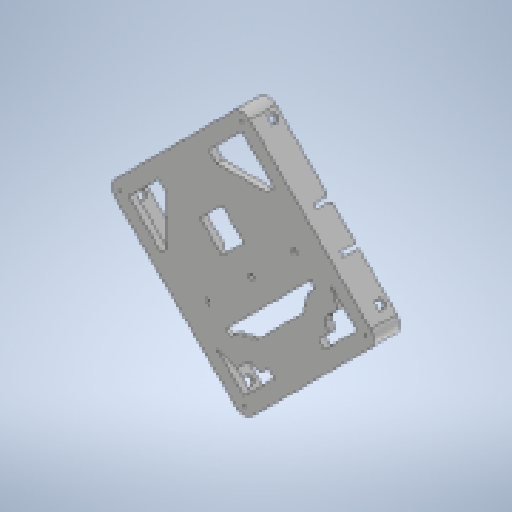
# Autodesk Inventor part: RobotStandBase
Saved by Autodesk Inventor 2025.1 (Build 291241000, 241)
## iProperties
Created: 2026-05-10
Part Number: RobotStandBase
Material: Generic
Document SubType Name: Modeling
Designer: User
Density: 1 g/cm^3
Appearance: Default
Author: User
## iProperties of the stored document RobotStandBase_3DPrint.ipt
Created: 2026-05-10
Part Number: RobotStandBase_3DPrint
Material: Generic
Document SubType Name: Modeling
Designer: User
Density: 1 g/cm^3
Appearance: Default
Author: User
Autodesk Inventor part; units mm, degrees
(part 1 of 2)
ref_plane "YZ Plane" through (0, 0, 0) normal (1, 0, 0) x (0, 1, 0)
ref_plane "XZ Plane" through (0, 0, 0) normal (0, 1, 0) x (-1, 0, 0)
ref_plane "XY Plane" through (0, 0, 0) normal (0, 0, 1) x (1, 0, 0)
sketch "Sketch1" plane through (0, 0, 0) normal (0, 0, 1) x (1, 0, 0)
  line L0 (-56.2755, 56.2755) -> (-1.1212, 1.1212) projected
  line L1 (-1.1163, -113.435) -> (-56.398, -168.7168) projected
  line L2 (-167.8767, -165.6343) -> (-223.031, -110.4799) projected
  line L3 (-226.1086, 0.9938) -> (-170.8268, 56.2755) projected
  line L4 (-280.3067, -53.2043) -> (-226.1086, 0.9938)
  line L5 (-280.3067, -53.2043) -> (-223.031, -110.4799)
  line L6 (-170.8268, 56.2755) -> (-113.5512, 113.5512)
  line L7 (-113.5512, 113.5512) -> (-56.2755, 56.2755)
  line L8 (-1.1212, 1.1212) -> (56.1594, -56.1594)
  line L9 (56.1594, -56.1594) -> (-1.1163, -113.435)
  line L10 (-167.8767, -165.6343) -> (-110.5961, -222.9149)
  line L11 (-56.398, -168.7168) -> (-110.5961, -222.9149)
  point P0 (0, 0)
  constraints: 16 end point, 4 point on line, 2 perpendicular, 1 collinear
extrude "Extrusion1" add sketch "Sketch1" along normal blind 5
sketch "Sketch2" plane through (0, 0, 0) normal (0, 0, -1) x (-1, 0, 0)
  line L0 (-56.1594, -56.1594) -> (113.5512, 113.5512) projected
  line L1 (-52.6239, -59.6949) -> (117.0867, 110.0157)
  line L2 (113.5512, 113.5512) -> (280.3067, -53.2043) projected
  line L3 (110.5961, -222.9149) -> (-56.1594, -56.1594) projected
  point P0 (0, 0)
  dimension "d2" = 5
  constraints: 2 end point, 1 parallel
  measures "d2" distance between parallel lines of L0 L1
ref_plane "Work Plane1" through (-173.6553, -9.9637, -27.5) normal (0, 0, 1) x (1, 0, 0)
extrude "Extrusion2" add sketch "Sketch2" along normal up to surface (27.5 mm away)
sketch "Sketch3" plane through (-113.5512, 113.5512, -27.5) normal (0.7071068, 0.7071068, 0) x (-0.7071068, 0.7071068, 0)
  line L0 (-106.0221, 0) -> (-106.0221, 18.3301) projected
  line L1 (-111.0221, 18.3301) -> (-111.0221, 0) projected
  line L2 (-106.0221, 18.3301) -> (-111.0221, 18.3301) projected
  line L3 (-154, 0) -> (-154, 18.3301) projected
  line L4 (-159, 18.3301) -> (-159, -12) projected
  line L5 (-154, 18.3301) -> (-159, 18.3301) projected
  line L6 (-111.2221, 0) -> (-111.2221, 18.5301)
  line L7 (-111.2221, 18.5301) -> (-105.8221, 18.5301)
  line L8 (-105.8221, 18.5301) -> (-105.8221, 0)
  line L9 (-153.8, 0) -> (-153.8, 18.5301)
  line L10 (-153.8, 18.5301) -> (-159.2, 18.5301)
  line L11 (-159.2, 18.5301) -> (-159.2, -12)
  line L12 (0, 0) -> (-240.007, 0) projected
  point P0 (-160.5856, 27.5)
  point P1 (-159.2, 0)
  dimension "d5" = 0.2
  dimension "d6" = 0.2
  constraints: 12 end point, 4 other
  measures "d5" distance between parallel lines of L1 L6
  measures "d6" distance between parallel lines of L3 L9
extrude "Extrusion3" cut sketch "Sketch3" against normal blind 10
sketch "Sketch4" plane through (0, 0, 0) normal (0, 0, -1) x (-1, 0, 0)
  line L0 (280.3067, -53.2043) -> (110.5961, -222.9149) projected
  line L1 (276.7711, -49.6687) -> (107.0605, -219.3793)
  line L2 (107.0605, -219.3793) -> (110.5961, -222.9149)
  line L3 (117.0867, 110.0157) -> (280.3067, -53.2043) projected
  line L4 (276.7711, -49.6687) -> (280.3067, -53.2043)
  line L5 (110.5961, -222.9149) -> (-52.6239, -59.6949) projected
  point P0 (0, 0)
  dimension "d9" = 5
  constraints: 6 end point, 1 collinear, 1 parallel
  measures "d9" distance between parallel lines of L0 L1
ref_plane "Work Plane2" through (-226.1086, -128.1732, -27.5) normal (0, 0, 1) x (1, 0, 0)
extrude "Extrusion4" add sketch "Sketch4" along normal up to surface (27.5 mm away)
sketch "Sketch5" plane through (-110.5961, -222.9149, 5) normal (-0.7071068, -0.7071068, 0) x (-0.7071068, 0.7071068, 0)
  line L0 (81.007, 14.1699) -> (81.007, 44.5) projected
  line L1 (86.007, 14.1699) -> (86.007, 32.5) projected
  line L2 (81.007, 14.1699) -> (86.007, 14.1699) projected
  line L3 (128.9849, 32.5) -> (128.9849, 14.1699) projected
  line L4 (128.9849, 14.1699) -> (133.9849, 14.1699) projected
  line L5 (133.9849, 14.1699) -> (133.9849, 32.5) projected
  line L6 (86.207, 32.5) -> (86.207, 13.9699)
  line L7 (86.207, 13.9699) -> (80.807, 13.9699)
  line L8 (80.807, 13.9699) -> (80.807, 44.5)
  line L9 (128.7849, 32.5) -> (128.7849, 13.9699)
  line L10 (128.7849, 13.9699) -> (134.1849, 13.9699)
  line L11 (134.1849, 13.9699) -> (134.1849, 32.5)
  line L12 (0, 32.5) -> (240.007, 32.5) projected
  point P0 (79.4214, 5)
  point P1 (80.807, 32.5)
  dimension "d12" = 0.2
  dimension "d13" = 0.2
  constraints: 12 end point, 4 other
  measures "d12" distance between parallel lines of L1 L6
  measures "d13" distance between parallel lines of L3 L9
extrude "Extrusion5" cut sketch "Sketch5" against normal blind 10
sketch "Sketch6" plane through (0, 0, 0) normal (0, 0, -1) x (-1, 0, 0)
  line L0 (107.0605, -219.3793) -> (-52.6239, -59.6949) projected
  line L1 (110.5961, -215.8438) -> (-49.0883, -56.1594)
  line L2 (117.0867, 110.0157) -> (-52.6239, -59.6949) projected
  line L3 (107.0605, -219.3793) -> (276.7711, -49.6687) projected
  point P0 (0, 0)
  dimension "d16" = 5
  constraints: 2 end point, 1 parallel
  measures "d16" distance between parallel lines of L0 L1
extrude "Extrusion6" add sketch "Sketch6" along normal up to surface (27.5 mm away)
sketch "Sketch7" plane through (56.1594, -56.1594, 5) normal (0.7071068, -0.7071068, 0) x (-0.7071068, -0.7071068, 0)
  line L0 (91, 32.5) -> (91, 14.1699) projected
  line L1 (96, 14.1699) -> (96, 32.5) projected
  line L2 (91, 14.1699) -> (96, 14.1699) projected
  line L3 (144.1802, 32.5) -> (144.1802, 14.1699) projected
  line L4 (144.1802, 14.1699) -> (149.1802, 14.1699) projected
  line L5 (149.1802, 14.1699) -> (149.1802, 32.5) projected
  line L6 (90.8, 32.5) -> (90.8, 13.9699)
  line L7 (90.8, 13.9699) -> (96.2, 13.9699)
  line L8 (96.2, 13.9699) -> (96.2, 32.5)
  line L9 (143.9802, 32.5) -> (143.9802, 13.9699)
  line L10 (143.9802, 13.9699) -> (149.3802, 13.9699)
  line L11 (149.3802, 13.9699) -> (149.3802, 32.5)
  line L12 (0, 32.5) -> (235.8278, 32.5) projected
  point P0 (0, 5)
  dimension "d19" = 0.2
  dimension "d20" = 0.2
  constraints: 12 end point, 5 other
  measures "d19" distance between parallel lines of L0 L6
  measures "d20" distance between parallel lines of L3 L9
extrude "Extrusion7" cut sketch "Sketch7" against normal blind 10
sketch "Sketch8" plane through (0, 0, 0) normal (0, 0, -1) x (-1, 0, 0)
  line L0 (117.0867, 110.0157) -> (276.7711, -49.6687) projected
  line L1 (113.5512, 106.4801) -> (273.2356, -53.2043)
  line L2 (117.0867, 110.0157) -> (-49.0883, -56.1594) projected
  line L3 (110.5961, -215.8438) -> (276.7711, -49.6687) projected
  point P0 (0, 0)
  dimension "d23" = 5
  constraints: 2 end point, 1 parallel
  measures "d23" distance between parallel lines of L0 L1
extrude "Extrusion8" add sketch "Sketch8" along normal up to surface (27.5 mm away)
sketch "Sketch9" plane through (-280.3067, -53.2043, -27.5) normal (-0.7071068, 0.7071068, 0) x (-0.7071068, -0.7071068, 0)
  line L0 (-139.8278, 0) -> (-139.8278, 18.3301) projected
  line L1 (-150.8278, 0) -> (-144.8278, 6) projected
  line L2 (-144.8278, 18.3301) -> (-144.8278, 6) projected
  line L3 (-139.8278, 18.3301) -> (-144.8278, 18.3301) projected
  line L4 (-91.6476, 18.3301) -> (-91.6476, 0) projected
  line L5 (-86.6476, 6) -> (-80.6476, 0) projected
  line L6 (-86.6476, 6) -> (-86.6476, 18.3301) projected
  line L7 (-86.6476, 18.3301) -> (-91.6476, 18.3301) projected
  line L8 (-91.8476, 0) -> (-91.8476, 18.5301)
  line L9 (-91.8476, 18.5301) -> (-86.4476, 18.5301)
  line L10 (-86.4476, 18.5301) -> (-86.4476, 6.0828)
  line L11 (-86.4476, 6.0828) -> (-80.5062, 0.1414)
  line L12 (-139.6278, 0) -> (-139.6278, 18.5301)
  line L13 (-139.6278, 18.5301) -> (-145.0278, 18.5301)
  line L14 (-145.0278, 18.5301) -> (-145.0278, 6.0828)
  line L15 (-145.0278, 6.0828) -> (-150.9693, 0.1414)
  line L16 (-230.8278, 0) -> (-5, 0) projected
  line L17 (-145.0278, 6.0828) -> (-151.1107, 0)
  line L18 (-86.4476, 6.0828) -> (-80.3648, 0)
  point P0 (-235.8278, 27.5)
  point P1 (-150.9693, 0.1414)
  point P2 (-80.5062, 0.1414)
  dimension "d26" = 0.2
  dimension "d27" = 0.2
  constraints: 20 end point, 2 point on line, 9 other
  measures "d26" distance between parallel lines of L4 L8
  measures "d27" distance between parallel lines of L0 L12
extrude "Extrusion9" cut sketch "Sketch9" against normal blind 10
chamfer "Chamfer1" distance 2 angle 45 16 edges at (-221.7124, 1.8544, -27.5) (-213.5928, 9.974, -27.5) (-179.8071, 43.7597, -27.5) (-171.6875, 51.8793, -27.5) (-36.673, 33.1375, -27.5) (-40.4914, 36.9559, -27.5) (-6.5659, 3.0304, -27.5) (-2.7476, -0.788, -27.5) (-13.632, -122.4153, -27.5) (-9.8137, -118.5969, -27.5) (-47.4178, -156.201, -27.5) (-51.2361, -160.0194, -27.5) (-165.9675, -164.0079, -27.5) (-169.7859, -160.1895, -27.5) (-199.893, -130.0824, -27.5) (-203.7113, -126.2641, -27.5)
fillet "Fillet1" radius 9 4 edges at (49.0883, -56.1594, -13.75) (-273.2356, -53.2043, -13.75) (-113.5512, 106.4801, -13.75) (-110.5961, -215.8438, -13.75)
fillet "Fillet2" radius 14 4 edges at (-110.5961, -222.9149, -11.25) (-280.3067, -53.2043, -11.25) (56.1594, -56.1594, -11.25) (-113.5512, 113.5512, -11.25)
chamfer "Chamfer2" distance 9 angle 45 8 edges at (-32.2314, 25.1604, 0) (45.3604, -56.1594, 0) (-30.7539, -136.0016, 0) (-110.5961, -212.1159, 0) (-191.9158, -134.524, 0) (-269.5077, -53.2043, 0) (-193.3934, 26.6379, 0) (-113.5512, 102.7522, 0)
sketch "Sketch10" plane through (-38.4408, 31.3697, -9) normal (-0.7071068, -0.7071068, 0) x (-0.7071068, 0.7071068, 0)
  line L0 (-42.5779, 16.5) -> (-42.5779, 0) projected
  line L1 (-47.9779, 0) -> (-47.9779, 16.5) projected
  line L2 (-49.9779, 18.5) -> (-47.9779, 16.5) projected
  line L3 (-42.5779, 16.5) -> (-40.5779, 18.5) projected
  line L4 (-40.5779, 18.5) -> (-2, 18.5) projected
  line L5 (-114.7849, 18.5) -> (-49.9779, 18.5) projected
  line L6 (-42.5779, -0.0301) -> (-47.9779, -0.0301) projected
  line L7 (-2, 18.5) -> (0, 16.5) projected
  line L8 (5.4, 16.5) -> (7.4, 18.5) projected
  line L9 (7.4, 18.5) -> (97.2221, 18.5) projected
  line L10 (5.4, 16.5) -> (5.4, 0) projected
  line L11 (5.4, -0.0301) -> (0, -0.0301) projected
  line L12 (0, 0) -> (0, 16.5) projected
  line L13 (-3, 0) -> (-3, 15.2574)
  line L14 (-3, 15.2574) -> (-3.2426, 15.5)
  line L15 (-3.2426, 15.5) -> (-39.3352, 15.5)
  line L16 (-39.3352, 15.5) -> (-39.5779, 15.2574)
  line L17 (-39.5779, 15.2574) -> (-39.5779, 0)
  line L18 (-50.9779, 0) -> (-50.9779, 15.2574)
  line L19 (-50.9779, 15.2574) -> (-51.2205, 15.5)
  line L20 (-51.2205, 15.5) -> (-114.7849, 15.5)
  line L21 (8.4, 0) -> (8.4, 15.2574)
  line L22 (8.4, 15.2574) -> (8.6426, 15.5)
  line L23 (8.6426, 15.5) -> (97.2221, 15.5)
  line L24 (-39.5779, 18.5) -> (-39.5779, 0)
  line L25 (0, 0) -> (-42.5779, 0) projected
  line L26 (-39.5779, 0) -> (-39.5779, -3)
  line L27 (-39.5779, -3) -> (-50.9779, -3)
  line L28 (-50.9779, -3) -> (-50.9779, 18.5)
  line L29 (-3, 18.5) -> (-3, 0)
  line L30 (-3, 0) -> (-3, -3)
  line L31 (-3, 0) -> (0, 0) construction
  line L32 (-3, -3) -> (8.4, -3)
  line L33 (8.4, -3) -> (8.4, 18.5)
  line L34 (5.4, -0.0301) -> (5.4, 0) projected
  line L35 (0, 0) -> (0, -0.0301) projected
  line L36 (-47.9779, 0) -> (-47.9779, -0.0301) projected
  line L37 (-42.5779, -0.0301) -> (-42.5779, 0) projected
  point P0 (-49.3635, -9)
  point P1 (-3, 15.2574)
  point P2 (8.4, 0)
  point P3 (8.4, 15.2574)
  point P4 (-50.9779, 15.2574)
  point P5 (-50.9779, 0)
  point P6 (-39.5779, 15.2574)
  dimension "d174" = 1
  dimension "d38" = 3
  dimension "d39" = 3
  dimension "d40" = 3
  dimension "d41" = 3
  dimension "d42" = 90
  dimension "d43" = 3
  dimension "d44" = 90
  dimension "d45" = 90
  constraints: 40 end point, 7 point on line, 2 perpendicular, 1 collinear, 1 horizontal, 1 vertical, 8 other
  measures "d38" distance between parallel lines of L12 L13
  measures "d39" distance between parallel lines of L1 L18
  measures "d40" distance between parallel lines of L10 L21
  measures "d41" distance of L17.end L26.end
  measures "d42" angle of L26 L27
  measures "d43" distance of L13.start L30.end
  measures "d44" angle of L30 L31
  measures "d45" angle of L32 L30
extrude "Extrusion10" add sketch "Sketch10" along normal blind 3 contours L3 L4 L24 L17 L25 L0 | L25 L26 L27 L28 L18 L5 L2 L1 L36 L6 L37 | L13 L29 L4 L7 L12 L25 | L25 L35 L11 L34 L10 L8 L9 L33 L21 L32 L30
sketch "Sketch11" plane through (-49.4684, -161.7872, -8.9699) normal (0.7071068, -0.7071068, 0) x (-0.7071068, -0.7071068, 0)
  line L0 (-135.3802, -13.9699) -> (-135.3802, 18.5301) projected
  line L1 (72.4476, -13.9699) -> (-135.3802, -13.9699) projected
  line L2 (72.4476, 18.5301) -> (72.4476, -13.9699) projected
  line L3 (2, 18.5301) -> (72.4476, 18.5301) projected
  line L4 (0, 16.5301) -> (2, 18.5301) projected
  line L5 (0, 16.5301) -> (0, 0) projected
  line L6 (0, 0) -> (-5.4, 0) projected
  line L7 (-5.4, 0) -> (-5.4, 16.5301) projected
  line L8 (-7.4, 18.5301) -> (-5.4, 16.5301) projected
  line L9 (-51.1802, 18.5301) -> (-7.4, 18.5301) projected
  line L10 (-53.1802, 16.5301) -> (-51.1802, 18.5301) projected
  line L11 (-53.1802, 16.5301) -> (-53.1802, 0) projected
  line L12 (-53.1802, 0) -> (-58.5802, 0) projected
  line L13 (-58.5802, 0) -> (-58.5802, 16.5301) projected
  line L14 (-60.5802, 18.5301) -> (-58.5802, 16.5301) projected
  line L15 (-135.3802, 18.5301) -> (-60.5802, 18.5301) projected
  line L16 (-61.8229, 15.5301) -> (-61.5802, 15.2875)
  line L17 (-61.5802, 15.2875) -> (-61.5802, -3)
  line L18 (-61.5802, -3) -> (-50.1802, -3)
  line L19 (-50.1802, -3) -> (-50.1802, 15.2875)
  line L20 (-50.1802, 15.2875) -> (-49.9376, 15.5301)
  line L21 (-49.9376, 15.5301) -> (-8.6426, 15.5301)
  line L22 (-8.6426, 15.5301) -> (-8.4, 15.2875)
  line L23 (-8.4, 15.2875) -> (-8.4, -3)
  line L24 (-8.4, -3) -> (3, -3)
  line L25 (3, -3) -> (3, 15.2875)
  line L26 (3, 15.2875) -> (3.2426, 15.5301)
  line L27 (3.2426, 15.5301) -> (69.4476, 15.5301)
  line L28 (69.4476, 15.5301) -> (69.4476, -10.9699)
  line L29 (69.4476, -10.9699) -> (-132.3802, -10.9699)
  line L30 (-132.3802, -10.9699) -> (-132.3802, 15.5301)
  line L31 (-132.3802, 15.5301) -> (-61.8229, 15.5301)
  line L32 (-61.5802, -3) -> (-61.5802, 18.5301)
  line L33 (-50.1802, -3) -> (-50.1802, 18.5301)
  line L34 (-51.1802, 18.5301) -> (-7.4, 18.5301) projected
  line L35 (-8.4, -3) -> (-8.4, 18.5301)
  line L36 (3, -3) -> (3, 18.5301)
  point P0 (-149.3802, -8.9699)
  point P1 (-8.4, 15.2875)
  point P2 (3, 15.2875)
  point P3 (-61.5802, 15.2875)
  point P4 (-50.1802, 15.2875)
  point P5 (-50.1802, 18.5301)
  dimension "d48" = 3
  constraints: 40 end point, 4 point on line, 2 parallel, 1 perpendicular, 1 vertical, 15 other
  measures "d48" distance between parallel lines of L15 L31
extrude "Extrusion11" add sketch "Sketch11" against normal blind 8 contours L15 L14 L13 L12 L11 L10 L9 L33 L19 L18 L17 L32 | L36 L25 L24 L23 L35 L9 L8 L7 L6 L5 L4 L3
sketch "Sketch12" plane through (-205.4791, -128.0318, -8.9699) normal (-0.7071068, -0.7071068, 0) x (-0.7071068, 0.7071068, 0)
  line L0 (91.8221, 18.5301) -> (91.8221, -13.9699) projected
  line L1 (2, 18.5301) -> (91.8221, 18.5301) projected
  line L2 (0, 16.5301) -> (2, 18.5301) projected
  line L3 (0, 16.5301) -> (0, 0) projected
  line L4 (0, 0) -> (-5.4, 0) projected
  line L5 (-5.4, 0) -> (-5.4, 16.5301) projected
  line L6 (-7.4, 18.5301) -> (-5.4, 16.5301) projected
  line L7 (-45.9779, 18.5301) -> (-7.4, 18.5301) projected
  line L8 (-47.9779, 16.5301) -> (-45.9779, 18.5301) projected
  line L9 (-47.9779, 16.5301) -> (-47.9779, 0) projected
  line L10 (-47.9779, 0) -> (-53.3779, 0) projected
  line L11 (-53.3779, 0) -> (-53.3779, 16.5301) projected
  line L12 (-55.3779, 18.5301) -> (-53.3779, 16.5301) projected
  line L13 (-120.1849, 18.5301) -> (-55.3779, 18.5301) projected
  line L14 (-120.1849, -13.9699) -> (-120.1849, 18.5301) projected
  line L15 (91.8221, -13.9699) -> (-120.1849, -13.9699) projected
  line L16 (-8.4, 15.2875) -> (-8.4, -3)
  line L17 (-8.4, -3) -> (3, -3)
  line L18 (3, -3) -> (3, 15.2875)
  line L19 (3, 15.2875) -> (3.2426, 15.5301)
  line L20 (3.2426, 15.5301) -> (88.8221, 15.5301)
  line L21 (88.8221, 15.5301) -> (88.8221, -10.9699)
  line L22 (88.8221, -10.9699) -> (-117.1849, -10.9699)
  line L23 (-117.1849, -10.9699) -> (-117.1849, 15.5301)
  line L24 (-117.1849, 15.5301) -> (-56.6205, 15.5301)
  line L25 (-56.6205, 15.5301) -> (-56.3779, 15.2875)
  line L26 (-56.3779, 15.2875) -> (-56.3779, -3)
  line L27 (-56.3779, -3) -> (-44.9779, -3)
  line L28 (-44.9779, -3) -> (-44.9779, 15.2875)
  line L29 (-44.9779, 15.2875) -> (-44.7352, 15.5301)
  line L30 (-44.7352, 15.5301) -> (-8.6426, 15.5301)
  line L31 (-8.6426, 15.5301) -> (-8.4, 15.2875)
  line L32 (3, 18.5301) -> (3, 0.0301) projected
  line L33 (3, -3) -> (3, 18.5301)
  line L34 (-8.4, -3) -> (-8.4, 18.5301)
  line L35 (-44.9779, 0.0301) -> (-44.9779, -2.9699) projected
  line L36 (-44.9779, 18.5301) -> (-44.9779, 0.0301) projected
  line L37 (-44.9779, -2.9699) -> (-44.9779, 18.5301)
  line L38 (-56.3779, -3) -> (-56.3779, 18.5301)
  point P0 (-54.7635, -8.9699)
  point P1 (-56.3779, 15.2875)
  point P2 (-8.4, 15.2875)
  dimension "d51" = 3
  constraints: 40 end point, 3 point on line, 1 collinear, 1 perpendicular, 15 other
  measures "d51" distance between parallel lines of L5 L16
extrude "Extrusion12" add sketch "Sketch12" against normal blind 8 contours L32 L18 L17 L16 L34 L7 L6 L5 L4 L3 L2 L1 | L13 L12 L11 L10 L9 L8 L7 L36 L28 L27 L26 L38
sketch "Sketch13" plane through (-177.7565, 49.3459, -21.4172) normal (-0.7071068, 0.7071068, 0) x (-0.7071068, -0.7071068, 0)
  line L0 (-76.8, -6.0828) -> (-76.8, 26.4172) projected
  line L1 (-8.0828, -6.0828) -> (-76.8, -6.0828) projected
  line L2 (-4.6686, -4.6686) -> (-8.0828, -6.0828) projected
  line L3 (-4.6686, -4.6686) -> (0, 0) projected
  line L4 (0, 0) -> (0, 12.4473) projected
  line L5 (0, 12.4473) -> (5.4, 12.4473) projected
  line L6 (5.4, 12.4473) -> (5.4, -4.0828) projected
  line L7 (7.4, -6.0828) -> (5.4, -4.0828) projected
  line L8 (51.1802, -6.0828) -> (7.4, -6.0828) projected
  line L9 (53.1802, -4.0828) -> (51.1802, -6.0828) projected
  line L10 (53.1802, -4.0828) -> (53.1802, 12.4473) projected
  line L11 (53.1802, 12.4473) -> (58.5802, 12.4473) projected
  line L12 (58.5802, 12.4473) -> (58.5802, 0) projected
  line L13 (58.5802, 0) -> (63.2489, -4.6686) projected
  line L14 (66.6631, -6.0828) -> (63.2489, -4.6686) projected
  line L15 (131.0278, -6.0828) -> (66.6631, -6.0828) projected
  line L16 (131.0278, 26.4172) -> (131.0278, -6.0828) projected
  line L17 (-76.8, 26.4172) -> (131.0278, 26.4172) projected
  line L18 (8.6426, -3.0828) -> (8.4, -2.8402)
  line L19 (8.4, -2.8402) -> (8.4, 15.4473)
  line L20 (8.4, 15.4473) -> (-3, 15.4473)
  line L21 (-3, 15.4473) -> (-3, 1.2426)
  line L22 (-3, 1.2426) -> (-6.368, -2.1254)
  line L23 (-6.368, -2.1254) -> (-8.6796, -3.0828)
  line L24 (-8.6796, -3.0828) -> (-73.8, -3.0828)
  line L25 (-73.8, -3.0828) -> (-73.8, 23.4172)
  line L26 (-73.8, 23.4172) -> (128.0278, 23.4172)
  line L27 (128.0278, 23.4172) -> (128.0278, -3.0828)
  line L28 (128.0278, -3.0828) -> (67.2598, -3.0828)
  line L29 (67.2598, -3.0828) -> (64.9482, -2.1254)
  line L30 (64.9482, -2.1254) -> (61.5802, 1.2426)
  line L31 (61.5802, 1.2426) -> (61.5802, 15.4473)
  line L32 (61.5802, 15.4473) -> (50.1802, 15.4473)
  line L33 (50.1802, 15.4473) -> (50.1802, -2.8402)
  line L34 (50.1802, -2.8402) -> (49.9376, -3.0828)
  line L35 (49.9376, -3.0828) -> (8.6426, -3.0828)
  line L36 (50.1802, 15.4172) -> (50.1802, -6.0828) projected
  line L37 (50.1802, 15.4473) -> (50.1802, -6.0828)
  line L38 (8.4, -6.0828) -> (8.4, 15.4172) projected
  line L39 (8.4, 15.4473) -> (8.4, -6.0828)
  line L40 (-8.6796, -3.0828) -> (-8.6796, -6.0828)
  line L41 (67.2598, -3.0828) -> (67.2598, -6.0828)
  point P0 (-90.8, 21.4172)
  dimension "d54" = 3
  constraints: 44 end point, 2 point on line, 1 parallel, 1 perpendicular, 17 other
  measures "d54" distance between parallel lines of L8 L35
extrude "Extrusion13" add sketch "Sketch13" against normal blind 8 contours L40 L23 L22 L21 L20 L19 L38 L8 L7 L6 L5 L4 L3 L2 L1 | L15 L14 L13 L12 L11 L10 L9 L8 L36 L33 L32 L31 L30 L29 L41
sketch "Sketch14" plane through (0, 0, 0) normal (0, 0, -1) x (-1, 0, 0)
  line L0 (168.0234, -127.9604) -> (169.6482, -127.3987) projected
  line L1 (169.6482, -127.3987) -> (173.5542, -123.4928) projected
  line L2 (173.5542, -123.4928) -> (171.3554, -97.3754) projected
  line L3 (171.3554, -97.3754) -> (171.5721, -97.1586) projected
  line L4 (69.9473, 4.4661) -> (171.5721, -97.1586) projected
  line L5 (69.9473, 4.4661) -> (40.9763, 6.9046) projected
  line L6 (40.9763, 6.9046) -> (37.0674, 2.9956) projected
  line L7 (37.0674, 2.9956) -> (27.3005, -25.3557) projected
  line L8 (27.3005, -25.3557) -> (27.2484, -25.4078) projected
  line L9 (27.2484, -25.4078) -> (139.62, -137.7795) projected
  line L10 (139.62, -137.7795) -> (139.6721, -137.7273) projected
  line L11 (139.6721, -137.7273) -> (168.0234, -127.9604) projected
  line L12 (139.6721, -137.7273) -> (171.5721, -97.1586)
  line L13 (27.2484, -25.4078) -> (69.9473, 4.4661)
  line L14 (83.4342, -81.5936) -> (119.7206, -45.3072)
  circle A0 centre (155.6221, -117.443) radius 1.5
  circle A1 centre (101.5774, -63.4504) radius 1.5
  circle A2 centre (48.5978, -10.4708) radius 1.5
  circle A3 centre (48.5978, -10.4708) radius 1.5 projected
  circle A4 centre (101.5774, -63.4504) radius 1.5 projected
  circle A5 centre (155.6221, -117.443) radius 1.5 projected
  point P0 (0, 0)
  dimension "d57" = 3
  dimension "d58" = 3
  dimension "d59" = 3
  constraints: 6 end point, 4 midpoint, 3 centre point, 1 perpendicular, 1 point on line
  measures "d57" diameter of A0
  measures "d58" diameter of A1
  measures "d59" diameter of A2
extrude "Extrusion14" cut sketch "Sketch14" against normal blind 8 contours A0 L12 | L12 A0 | A1 L14 | L14 A1 | A2 L13 | L13 A2
sketch "Sketch15" plane through (0, 0, 5) normal (0, 0, 1) x (1, 0, 0)
  circle A0 centre (-48.5978, -10.4708) radius 1.5 projected
  circle A1 centre (-101.5774, -63.4504) radius 1.5 projected
  circle A2 centre (-155.6221, -117.443) radius 1.5 projected
  circle A3 centre (-155.6221, -117.443) radius 3.25
  circle A4 centre (-101.5774, -63.4504) radius 3.25
  circle A5 centre (-48.5978, -10.4708) radius 1.5 projected
  circle A6 centre (-48.5978, -10.4708) radius 3.25
  point P0 (0, 0)
  dimension "d62" = 6.5
  dimension "d63" = 6.5
  dimension "d64" = 6.5
  constraints: 3 centre point, 3 coincident
  measures "d62" diameter of A3
  measures "d63" diameter of A4
  measures "d64" diameter of A6
extrude "Extrusion15" cut sketch "Sketch15" against normal blind 3
sketch "Sketch16" plane through (-110.5961, -203.1159, -27.5) normal (0, 0, -1) x (-1, 0, 0)
  line L0 (51.4823, 38.7544) -> (6.364, -6.364) projected
  arc A0 (-6.364, -6.364) -> (6.364, -6.364) centre (0, 0) ccw projected
  line L1 (-6.364, -6.364) -> (-55.4708, 42.7429) projected
  line L2 (-55.4708, 42.7429) -> (-53.3495, 44.8642) projected
  line L3 (-54.0566, 45.5713) -> (-53.3495, 44.8642) projected
  line L4 (-59.7135, 39.9145) -> (-54.0566, 45.5713) projected
  line L5 (-59.7135, 39.9145) -> (-9.8995, -9.8995) projected
  arc A1 (-9.8995, -9.8995) -> (9.8995, -9.8995) centre (0, 0) ccw projected
  line L6 (9.8995, -9.8995) -> (55.725, 35.926) projected
  line L7 (55.725, 35.926) -> (50.0681, 41.5828) projected
  line L8 (49.361, 40.8757) -> (50.0681, 41.5828) projected
  line L9 (51.4823, 38.7544) -> (49.361, 40.8757) projected
  line L10 (-29.8223, 58.7748) -> (-54.198, 34.3991) projected
  line L11 (-45.5575, 38.7969) -> (-51.3488, 33.0057) projected
  line L12 (-44.8504, 38.0898) -> (-50.6417, 32.2986)
  line L13 (-50.6625, 37.9346) -> (-47.8341, 35.1062)
  line L14 (-47.8341, 35.1062) -> (-51.3696, 31.5706)
  line L15 (-51.3696, 31.5706) -> (-54.198, 34.3991)
  line L16 (-54.198, 34.3991) -> (-50.6625, 37.9346)
  line L17 (-85.1041, 114.0566) -> (-109.4798, 89.6808) projected
  line L18 (-95.7821, 107.6212) -> (-107.3585, 96.0448) projected
  line L19 (-101.136, 88.408) -> (-153.3204, 140.5925) projected
  line L20 (-156.856, 137.057) -> (-103.9644, 84.1654) projected
  line L21 (-107.3585, 96.0448) -> (-111.6011, 91.8021) projected
  line L22 (-112.3082, 92.5093) -> (-108.0656, 96.7519)
  line L23 (-108.0656, 96.7519) -> (-96.4892, 108.3283)
  line L24 (-108.7727, 96.0448) -> (-105.9443, 93.2164)
  line L25 (-105.9443, 93.2164) -> (-109.4798, 89.6808)
  line L26 (-109.4798, 89.6808) -> (-112.3082, 92.5093)
  line L27 (-112.3082, 92.5093) -> (-108.7727, 96.0448)
  point P0 (-110.5961, 203.1159)
  point P1 (-50.6417, 32.2986)
  point P2 (-112.3082, 92.5093)
  dimension "d67" = 1
  dimension "d68" = 1
  constraints: 22 end point, 8 point on line, 5 parallel, 2 perpendicular, 1 other
  measures "d67" distance between parallel lines of L11 L12
  measures "d68" distance between parallel lines of L21 L22
extrude "Extrusion16" cut sketch "Sketch16" against normal blind 2 contours L12 L14 L5 L10 L1 | L17 L20 L21 L19 | L21 L20 L22 L19
sketch "Sketch17" plane through (-205.4791, -128.0318, -8.9699) normal (-0.7071068, -0.7071068, 0) x (-0.7071068, 0.7071068, 0)
  arc A0 (78.6963, 12.5301) -> (86.9479, 12.5301) centre (82.8221, 9.3651) ccw projected
  circle A1 centre (82.8221, 9.3651) radius 5.2
  arc A2 (-100.0531, 9.3651) -> (-110.4531, 9.3651) centre (-105.2531, 9.3651) ccw projected
  point P0 (-54.7635, -8.9699)
  point P1 (86.9479, 12.5301)
  point P2 (78.6963, 12.5301)
  constraints: 1 centre point, 1 coincident, 1 concentric
extrude "Extrusion17" cut sketch "Sketch17" against normal through all
sketch "Sketch18" plane through (-205.4791, -128.0318, -8.9699) normal (-0.7071068, -0.7071068, 0) x (-0.7071068, 0.7071068, 0)
  circle A0 centre (-105.2531, 9.3651) radius 5.2 projected
  circle A1 centre (82.8221, 9.3651) radius 5.2 projected
  line L0 (77.6221, 4.1651) -> (88.0221, 4.1651)
  line L1 (88.0221, 4.1651) -> (88.0221, 9.3651)
  line L2 (77.6221, 4.1651) -> (77.6221, 9.3651)
  line L3 (-110.4531, 4.1651) -> (-100.0531, 4.1651)
  line L4 (-100.0531, 4.1651) -> (-100.0531, 9.3651)
  line L5 (-110.4531, 4.1651) -> (-110.4531, 9.3651)
  point P0 (-54.7635, -8.9699)
  point P1 (82.8221, 4.1651)
  point P2 (-105.2531, 4.1651)
  constraints: 12 end point, 4 point on circle, 3 tangent, 2 horizontal, 1 parallel
extrude "Extrusion18" cut sketch "Sketch18" against normal through all contours A0 | L4 L3 A0 | A0 L3 L5 | L1 L0 A1 | A1 L0 L2
sketch "Sketch19" plane through (0, 0, 0) normal (0, 0, -1) x (-1, 0, 0)
  line L0 (80.6463, 31.9048) -> (146.4561, 31.9048)
  line L1 (146.4561, 31.9048) -> (165.8771, 51.3258)
  line L2 (80.6463, 31.9048) -> (61.2253, 51.3258)
  line L3 (-36.3604, -56.1594) -> (113.5512, 93.7522) projected
  line L4 (113.5512, 93.7522) -> (260.5077, -53.2043) projected
  line L5 (201.6104, -23.5044) -> (221.1589, -3.956)
  line L6 (201.6104, -23.5044) -> (201.6104, -89.0593)
  line L7 (201.6104, -89.0593) -> (218.0813, -105.5302)
  line L8 (260.5077, -53.2043) -> (110.5961, -203.1159) projected
  line L9 (80.7737, -144.3411) -> (61.3478, -163.7671)
  line L10 (87.6903, -151.2576) -> (80.7737, -144.3411)
  line L11 (87.6903, -151.2576) -> (91.6237, -155.191)
  line L12 (91.6237, -155.191) -> (101.5016, -151.7881)
  line L13 (101.5016, -151.7881) -> (107.3644, -153.2088)
  line L14 (107.3644, -153.2088) -> (108.0393, -153.3992)
  ellipse E0 centre (95.5108, -186.7522) end of major axis (150.7623, -199.5036) minor radius 35.4384 (110.2496, -154.0628) -> (108.0393, -153.3992) ccw
  line L15 (121.0834, -164.8966) -> (110.2496, -154.0628)
  line L16 (143.4515, -157.164) -> (121.0834, -164.8966)
  line L17 (143.4515, -157.164) -> (155.3769, -161.0788)
  line L18 (143.4515, -157.164) -> (155.3769, -161.0788)
  line L19 (143.4515, -157.164) -> (155.3769, -161.0788)
  line L20 (110.5961, -203.1159) -> (-36.3604, -56.1594) projected
  line L21 (25.492, -89.0593) -> (6.066, -108.4853)
  line L22 (25.492, -89.0593) -> (15.5994, -79.1667)
  line L23 (11.6681, -75.2354) -> (15.5994, -79.1667)
  line L24 (15.0798, -65.3663) -> (11.6681, -75.2354)
  line L25 (13.6634, -59.5078) -> (15.0798, -65.3663)
  ellipse E1 centre (-19.8987, -71.3426) end of major axis (-32.6095, -16.1319) minor radius 35.4503 (13.4734, -58.8334) -> (12.8115, -56.6247) ccw
  line L26 (12.8115, -56.6247) -> (0.6153, -44.4285)
  line L27 (13.4734, -58.8334) -> (13.6634, -59.5078)
  line L28 (0.6153, -44.4285) -> (8.1231, -22.711)
  line L29 (4.4924, -10.8835) -> (8.1231, -22.711)
  line L30 (221.6168, -101.9946) -> (206.6104, -86.9882)
  line L31 (206.6104, -86.9882) -> (206.6104, -25.5755)
  line L32 (206.6104, -25.5755) -> (224.6944, -7.4915)
  line L33 (162.3416, 54.8613) -> (144.385, 36.9048)
  line L34 (144.385, 36.9048) -> (82.7174, 36.9048)
  line L35 (82.7174, 36.9048) -> (64.7608, 54.8613)
  line L36 (2.5305, -104.9498) -> (18.4209, -89.0593)
  line L37 (18.4209, -89.0593) -> (5.9203, -76.5587)
  line L38 (5.9203, -76.5587) -> (9.8756, -65.1173)
  line L39 (9.8756, -65.1173) -> (8.8254, -60.7736)
  line L40 (8.8254, -60.7736) -> (8.6633, -60.1983)
  line L41 (8.395, -59.2793) -> (-5.1325, -45.7518)
  line L42 (-5.1325, -45.7518) -> (2.8645, -22.6189)
  line L43 (2.8645, -22.6189) -> (-0.2875, -12.3507)
  line L44 (64.8833, -167.3026) -> (80.7737, -151.4122)
  line L45 (80.7737, -151.4122) -> (90.2977, -160.9361)
  line L46 (90.2977, -160.9361) -> (101.7465, -156.9921)
  line L47 (101.7465, -156.9921) -> (106.0961, -158.0462)
  line L48 (106.0961, -158.0462) -> (106.6721, -158.2087)
  line L49 (107.5941, -158.4784) -> (119.7601, -170.6444)
  line L50 (119.7601, -170.6444) -> (145.0852, -161.8896)
  line L51 (141.8921, -161.9145) -> (153.8174, -165.8294)
  line L52 (-29.2893, -56.1594) -> (113.5512, 86.6811)
  line L53 (113.5512, 86.6811) -> (253.4366, -53.2043)
  line L54 (253.4366, -53.2043) -> (110.5961, -196.0448)
  line L55 (110.5961, -196.0448) -> (-29.2893, -56.1594)
  spline S0 degree 3 poles (8.6633, -60.1983) (8.5756, -59.8914) (8.4862, -59.5851) (8.395, -59.2793) knots 0 0 0 0 1 1 1 1
  spline S1 degree 3 poles (106.6721, -158.2087) (106.98, -158.2969) (107.2873, -158.3868) (107.5941, -158.4784) knots 0 0 0 0 1 1 1 1
  point P0 (0, 0)
  point P1 (153.8563, 46.376)
  point P2 (73.2461, 46.376)
  point P3 (213.1315, -93.5094)
  point P4 (216.2091, -15.9768)
  point P5 (73.3686, -158.8173)
  point P6 (144.0258, -162.615)
  point P7 (143.4928, -162.44)
  point P8 (2.1319, -24.7381)
  point P9 (11.0157, -96.4645)
  dimension "d202" = 3
  dimension "d75" = 5
  dimension "d76" = 5
  dimension "d77" = 5
  dimension "d78" = 5
  dimension "d79" = 5
  dimension "d80" = 5
  constraints: 104 end point, 5 parallel, 1 horizontal, 1 vertical, 88 other
  measures "d75" distance between parallel lines of L6 L31
  measures "d76" distance between parallel lines of L0 L34
  measures "d77" distance between parallel lines of L24 L38
  measures "d78" distance between parallel lines of L15 L49
  measures "d79" distance between parallel lines of L17 L51
  measures "d80" distance between parallel lines of L20 L55
extrude "Extrusion19" cut sketch "Sketch19" against normal blind 10 contours L52 L53 L33 L34 L35 | L42 L41 S0 L40 L39 L38 L37 L36 L55 L52 | L53 L54 L30 L31 L32 | L44 L45 L46 L47 L48 S1 L49 L50 L51 L54 L55
sketch "Sketch20" plane through (0, 0, 0) normal (0, 0, -1) x (-1, 0, 0)
  line L0 (215.502, 11.6004) -> (144.8535, -59.0481)
  line L1 (177.8979, 49.2045) -> (107.2494, -21.4441)
  line L2 (181.4334, 45.6689) -> (110.7849, -24.9796)
  line L3 (219.0375, 8.0648) -> (148.389, -62.5837)
  line L4 (107.2494, -21.4441) -> (110.7849, -24.9796)
  line L5 (144.8535, -59.0481) -> (148.389, -62.5837)
  line L6 (174.3624, 52.74) -> (100.1783, -21.4441)
  line L7 (100.1783, -21.4441) -> (110.7849, -32.0507)
  line L8 (110.7849, -32.0507) -> (184.969, 42.1334)
  line L9 (211.9665, 15.1359) -> (137.7824, -59.0481)
  line L10 (137.7824, -59.0481) -> (148.389, -69.6548)
  line L11 (148.389, -69.6548) -> (222.5731, 4.5293)
  line L12 (137.7824, -59.0481) -> (110.7849, -32.0507)
  line L13 (110.7849, -32.0507) -> (137.7824, -5.0532)
  line L14 (137.7824, -5.0532) -> (164.7799, -32.0507)
  line L15 (164.7799, -32.0507) -> (137.7824, -59.0481)
  point P0 (0, 0)
  dimension "d202" = 3
  dimension "d83" = 5
  dimension "d84" = 5
  constraints: 32 end point, 3 equal length, 1 perpendicular, 16 other
  measures "d83" distance between parallel lines of L1 L6
  measures "d84" distance between parallel lines of L0 L9
extrude "Extrusion20" cut sketch "Sketch20" against normal blind 10
sketch "Sketch21" plane through (0, 0, 5) normal (0, 0, 1) x (1, 0, 0)
  arc A0 (-270.4072, -43.3048) -> (-270.4072, -63.1038) centre (-260.5077, -53.2043) ccw projected
  line L0 (-213.1315, -93.5094) -> (-253.4366, -53.2043) projected
  line L1 (-253.4366, -53.2043) -> (-216.2091, -15.9768) projected
  line L2 (-253.4366, -53.2043) -> (-274.5077, -53.2043)
  circle A1 centre (-263.9721, -53.2043) radius 1.5
  line L3 (-153.8563, 46.376) -> (-113.5512, 86.6811) projected
  line L4 (-113.5512, 86.6811) -> (-113.5512, 107.7522)
  arc A2 (-103.6517, 103.6517) -> (-123.4507, 103.6517) centre (-113.5512, 93.7522) ccw projected
  line L5 (-113.5512, 86.6811) -> (-92.4801, 86.6811) construction
  circle A3 centre (-113.5512, 97.2167) radius 1.5
  line L6 (29.2893, -56.1594) -> (-11.0157, -96.4645) projected
  line L7 (-2.1319, -24.7381) -> (29.2893, -56.1594) projected
  arc A4 (46.2599, -66.0589) -> (46.2599, -46.2599) centre (36.3604, -56.1594) ccw projected
  line L8 (29.2893, -56.1594) -> (50.3604, -56.1594)
  circle A5 centre (39.8249, -56.1594) radius 1.5
  line L9 (-110.5961, -196.0448) -> (-144.0258, -162.615) projected
  line L10 (-73.3686, -158.8173) -> (-110.5961, -196.0448) projected
  arc A6 (-120.4956, -213.0154) -> (-100.6966, -213.0154) centre (-110.5961, -203.1159) ccw projected
  line L11 (-110.5961, -196.0448) -> (-110.5961, -217.1159)
  circle A7 centre (-110.5961, -206.5803) radius 1.5
  point P0 (0, 0)
  dimension "d87" = 3
  dimension "d88" = 90
  dimension "d89" = 3
  dimension "d90" = 3
  dimension "d91" = 3
  constraints: 10 end point, 4 centre point, 4 midpoint, 4 point on circle, 1 horizontal, 1 perpendicular
  measures "d87" diameter of A1
  measures "d88" angle of L5 L4
  measures "d89" diameter of A3
  measures "d90" diameter of A5
  measures "d91" diameter of A7
extrude "Extrusion21" cut sketch "Sketch21" against normal through all
sketch "Sketch22" plane through (0, 0, 0) normal (0, 0, -1) x (-1, 0, 0)
  line L0 (2.1319, -24.7381) -> (-5.1325, -45.7518) projected
  line L1 (-5.1325, -45.7518) -> (8.395, -59.2793) projected
  line L2 (8.8254, -60.7736) -> (9.8756, -65.1173) projected
  circle A0 centre (-39.8249, -56.1594) radius 1.5 projected
  circle A1 centre (113.5512, 97.2167) radius 1.5 projected
  circle A2 centre (110.5961, -206.5803) radius 1.5 projected
  circle A3 centre (263.9721, -53.2043) radius 1.5 projected
  line L3 (164.7799, -32.0507) -> (137.7824, -5.0532) projected
  line L4 (137.7824, -5.0532) -> (110.7849, -32.0507) projected
  line L5 (110.7849, -32.0507) -> (137.7824, -59.0481) projected
  line L6 (137.7824, -59.0481) -> (164.7799, -32.0507) projected
  line L7 (213.1315, -93.5094) -> (253.4366, -53.2043) projected
  line L8 (253.4366, -53.2043) -> (216.2091, -15.9768) projected
  line L9 (216.2091, -15.9768) -> (206.6104, -25.5755) projected
  line L10 (206.6104, -25.5755) -> (206.6104, -86.9882) projected
  line L11 (206.6104, -86.9882) -> (213.1315, -93.5094) projected
  line L12 (106.6721, -158.2087) -> (106.0961, -158.0462) projected
  line L13 (106.0961, -158.0462) -> (101.7465, -156.9921) projected
  line L14 (101.7465, -156.9921) -> (90.2977, -160.9361) projected
  line L15 (90.2977, -160.9361) -> (80.7737, -151.4122) projected
  line L16 (80.7737, -151.4122) -> (73.3686, -158.8173) projected
  line L17 (73.3686, -158.8173) -> (110.5961, -196.0448) projected
  line L18 (110.5961, -196.0448) -> (144.0258, -162.615) projected
  line L19 (144.0258, -162.615) -> (143.4928, -162.44) projected
  line L20 (143.4928, -162.44) -> (119.7601, -170.6444) projected
  line L21 (119.7601, -170.6444) -> (107.5941, -158.4784) projected
  arc A4 (107.5941, -158.4784) -> (106.6721, -158.2087) centre (83.2615, -239.9478) ccw projected
  line L22 (153.8563, 46.376) -> (113.5512, 86.6811) projected
  line L23 (113.5512, 86.6811) -> (73.2461, 46.376) projected
  line L24 (73.2461, 46.376) -> (82.7174, 36.9048) projected
  line L25 (82.7174, 36.9048) -> (144.385, 36.9048) projected
  line L26 (144.385, 36.9048) -> (153.8563, 46.376) projected
  line L27 (2.1319, -24.7381) -> (-29.2893, -56.1594) projected
  line L28 (-29.2893, -56.1594) -> (11.0157, -96.4645) projected
  line L29 (11.0157, -96.4645) -> (18.4209, -89.0593) projected
  line L30 (18.4209, -89.0593) -> (5.9203, -76.5587) projected
  line L31 (5.9203, -76.5587) -> (9.8756, -65.1173) projected
  line L32 (9.8756, -65.1173) -> (8.8254, -60.7736) projected
  line L33 (8.8254, -60.7736) -> (8.6633, -60.1983) projected
  arc A5 (8.6633, -60.1983) -> (8.395, -59.2793) centre (-72.9104, -83.5196) ccw projected
  line L34 (8.395, -59.2793) -> (-5.1325, -45.7518) projected
  line L35 (-5.1325, -45.7518) -> (2.1319, -24.7381) projected
  circle A6 centre (155.6221, -117.443) radius 3.25 projected
  circle A7 centre (101.5774, -63.4504) radius 3.25 projected
  circle A8 centre (48.5978, -10.4708) radius 3.25 projected
  arc A9 (123.4507, 103.6517) -> (103.6517, 103.6517) centre (113.5512, 93.7522) ccw projected
  line L36 (123.4507, 103.6517) -> (270.4072, -43.3048) projected
  arc A10 (270.4072, -63.1038) -> (270.4072, -43.3048) centre (260.5077, -53.2043) ccw projected
  line L37 (270.4072, -63.1038) -> (120.4956, -213.0154) projected
  arc A11 (100.6966, -213.0154) -> (120.4956, -213.0154) centre (110.5961, -203.1159) ccw projected
  line L38 (100.6966, -213.0154) -> (-46.2599, -66.0589) projected
  arc A12 (-46.2599, -46.2599) -> (-46.2599, -66.0589) centre (-36.3604, -56.1594) ccw projected
  line L39 (-46.2599, -46.2599) -> (103.6517, 103.6517) projected
  line L40 (162.0784, -164.3615) -> (159.9571, -162.2401) projected
  line L41 (2.394, -4.6771) -> (4.5153, -6.7984) projected
  line L42 (159.9571, -162.2401) -> (4.5153, -6.7984)
  line L43 (80.7737, -113.888) -> (97.334, -130.4483)
  line L44 (97.334, -130.4483) -> (100.4472, -129.3758)
  line L45 (100.4472, -129.3758) -> (112.8262, -132.3755)
  line L46 (112.8262, -132.3755) -> (113.9248, -132.6856)
  arc A13 (121.9531, -135.3133) -> (113.9248, -132.6856) centre (83.2615, -239.9478) ccw
  line L47 (121.9531, -135.3133) -> (126.7824, -140.1425)
  line L48 (126.7824, -140.1425) -> (143.2738, -134.4415)
  line L49 (143.2738, -134.4415) -> (193.3009, -150.8641)
  line L50 (193.3009, -150.8641) -> (110.5961, -233.5689)
  line L51 (110.5961, -233.5689) -> (35.8445, -158.8173)
  line L52 (35.8445, -158.8173) -> (80.7737, -113.888)
  line L53 (36.5038, -66.3914) -> (35.3296, -69.788)
  line L54 (35.3296, -69.788) -> (54.601, -89.0593)
  line L55 (54.601, -89.0593) -> (11.0157, -132.6445)
  line L56 (11.0157, -132.6445) -> (-65.4694, -56.1594)
  line L57 (-65.4694, -56.1594) -> (62.618, 71.928)
  line L58 (62.618, 71.928) -> (24.2769, -38.9811)
  line L59 (24.2769, -38.9811) -> (30.7443, -45.4486)
  arc A14 (33.2756, -53.217) -> (30.7443, -45.4486) centre (-72.9104, -83.5196) ccw
  line L60 (33.2756, -53.217) -> (33.5798, -54.2971)
  line L61 (33.5798, -54.2971) -> (36.5038, -66.3914)
  line L62 (80.7737, -113.888) -> (35.6749, -68.7892)
  line L63 (80.7737, -113.888) -> (144.5531, -113.888) construction
  point P0 (0, 0)
  point P1 (135.0138, -137.2969)
  point P2 (27.4678, -29.7508)
  dimension "d202" = 3
  dimension "d94" = 26.5336
  dimension "d95" = 25.5832
  dimension "d96" = 135
  constraints: 44 end point, 4 point on circle, 2 centre point, 1 collinear, 1 equal length, 1 horizontal, 1 point on line, 19 other
  measures "d94" distance between parallel lines of L15 L43
  measures "d95" distance between parallel lines of L31 L53
  measures "d96" angle of L63 L62
extrude "Extrusion22" cut sketch "Sketch22" against normal blind 10 contours L42 L48 L47 A13 L46 L45 L44 L43 L62 L53 L61 L60 A14 L59 L58
sketch "Sketch23" plane through (0, 0, 0) normal (0, 0, -1) x (-1, 0, 0)
  line L0 (100.4472, -129.3758) -> (112.8262, -132.3755) projected
  line L1 (112.8262, -132.3755) -> (113.9248, -132.6856) projected
  arc A0 (121.9531, -135.3133) -> (113.9248, -132.6856) centre (83.2615, -239.9478) ccw projected
  line L2 (121.9531, -135.3133) -> (126.7824, -140.1425) projected
  line L3 (126.7824, -140.1425) -> (135.0138, -137.2969) projected
  line L4 (135.0138, -137.2969) -> (27.4678, -29.7508) projected
  line L5 (27.4678, -29.7508) -> (24.2769, -38.9811) projected
  line L6 (24.2769, -38.9811) -> (30.7443, -45.4486) projected
  arc A1 (33.2756, -53.217) -> (30.7443, -45.4486) centre (-72.9104, -83.5196) ccw projected
  line L7 (33.2756, -53.217) -> (33.5798, -54.2971) projected
  line L8 (33.5798, -54.2971) -> (36.5038, -66.3914) projected
  line L9 (36.5038, -66.3914) -> (35.6749, -68.7892) projected
  line L10 (35.6749, -68.7892) -> (97.334, -130.4483) projected
  line L11 (97.334, -130.4483) -> (100.4472, -129.3758) projected
  circle A2 centre (-39.8249, -56.1594) radius 1.5 projected
  circle A3 centre (113.5512, 97.2167) radius 1.5 projected
  circle A4 centre (110.5961, -206.5803) radius 1.5 projected
  circle A5 centre (263.9721, -53.2043) radius 1.5 projected
  line L12 (164.7799, -32.0507) -> (137.7824, -5.0532) projected
  line L13 (137.7824, -5.0532) -> (110.7849, -32.0507) projected
  line L14 (110.7849, -32.0507) -> (137.7824, -59.0481) projected
  line L15 (137.7824, -59.0481) -> (164.7799, -32.0507) projected
  line L16 (213.1315, -93.5094) -> (253.4366, -53.2043) projected
  line L17 (253.4366, -53.2043) -> (216.2091, -15.9768) projected
  line L18 (216.2091, -15.9768) -> (206.6104, -25.5755) projected
  line L19 (206.6104, -25.5755) -> (206.6104, -86.9882) projected
  line L20 (206.6104, -86.9882) -> (213.1315, -93.5094) projected
  line L21 (106.6721, -158.2087) -> (106.0961, -158.0462) projected
  line L22 (106.0961, -158.0462) -> (101.7465, -156.9921) projected
  line L23 (101.7465, -156.9921) -> (90.2977, -160.9361) projected
  line L24 (90.2977, -160.9361) -> (80.7737, -151.4122) projected
  line L25 (80.7737, -151.4122) -> (73.3686, -158.8173) projected
  line L26 (73.3686, -158.8173) -> (110.5961, -196.0448) projected
  line L27 (110.5961, -196.0448) -> (144.0258, -162.615) projected
  line L28 (144.0258, -162.615) -> (143.4928, -162.44) projected
  line L29 (143.4928, -162.44) -> (119.7601, -170.6444) projected
  line L30 (119.7601, -170.6444) -> (107.5941, -158.4784) projected
  arc A6 (107.5941, -158.4784) -> (106.6721, -158.2087) centre (83.2615, -239.9478) ccw projected
  line L31 (153.8563, 46.376) -> (113.5512, 86.6811) projected
  line L32 (113.5512, 86.6811) -> (73.2461, 46.376) projected
  line L33 (73.2461, 46.376) -> (82.7174, 36.9048) projected
  line L34 (82.7174, 36.9048) -> (144.385, 36.9048) projected
  line L35 (144.385, 36.9048) -> (153.8563, 46.376) projected
  line L36 (2.1319, -24.7381) -> (-29.2893, -56.1594) projected
  line L37 (-29.2893, -56.1594) -> (11.0157, -96.4645) projected
  line L38 (11.0157, -96.4645) -> (18.4209, -89.0593) projected
  line L39 (18.4209, -89.0593) -> (5.9203, -76.5587) projected
  line L40 (5.9203, -76.5587) -> (9.8756, -65.1173) projected
  line L41 (9.8756, -65.1173) -> (8.8254, -60.7736) projected
  line L42 (8.8254, -60.7736) -> (8.6633, -60.1983) projected
  arc A7 (8.6633, -60.1983) -> (8.395, -59.2793) centre (-72.9104, -83.5196) ccw projected
  line L43 (8.395, -59.2793) -> (-5.1325, -45.7518) projected
  line L44 (-5.1325, -45.7518) -> (2.1319, -24.7381) projected
  circle A8 centre (155.6221, -117.443) radius 3.25 projected
  circle A9 centre (101.5774, -63.4504) radius 3.25 projected
  circle A10 centre (48.5978, -10.4708) radius 3.25 projected
  arc A11 (123.4507, 103.6517) -> (103.6517, 103.6517) centre (113.5512, 93.7522) ccw projected
  line L45 (123.4507, 103.6517) -> (270.4072, -43.3048) projected
  arc A12 (270.4072, -63.1038) -> (270.4072, -43.3048) centre (260.5077, -53.2043) ccw projected
  line L46 (270.4072, -63.1038) -> (120.4956, -213.0154) projected
  arc A13 (100.6966, -213.0154) -> (120.4956, -213.0154) centre (110.5961, -203.1159) ccw projected
  line L47 (100.6966, -213.0154) -> (-46.2599, -66.0589) projected
  arc A14 (-46.2599, -46.2599) -> (-46.2599, -66.0589) centre (-36.3604, -56.1594) ccw projected
  line L48 (-46.2599, -46.2599) -> (103.6517, 103.6517) projected
  line L49 (145.2134, 34.9048) -> (81.889, 34.9048)
  line L50 (81.889, 34.9048) -> (70.4177, 46.376)
  line L51 (70.4177, 46.376) -> (113.5512, 89.5096)
  line L52 (113.5512, 89.5096) -> (156.6847, 46.376)
  line L53 (156.6847, 46.376) -> (145.2134, 34.9048)
  line L54 (204.6104, -87.8167) -> (204.6104, -24.7471)
  line L55 (204.6104, -24.7471) -> (216.2091, -13.1484)
  line L56 (216.2091, -13.1484) -> (256.265, -53.2043)
  line L57 (256.265, -53.2043) -> (213.1315, -96.3378)
  line L58 (213.1315, -96.3378) -> (204.6104, -87.8167)
  line L59 (-2.8334, -45.2225) -> (10.1648, -58.2207)
  arc A15 (10.5874, -59.6523) -> (10.1648, -58.2207) centre (-72.9104, -83.5196) ccw
  line L60 (10.5874, -59.6523) -> (10.7606, -60.2673)
  line L61 (10.7606, -60.2673) -> (11.9573, -65.2169)
  line L62 (11.9573, -65.2169) -> (8.2194, -76.0294)
  line L63 (8.2194, -76.0294) -> (21.2493, -89.0593)
  line L64 (21.2493, -89.0593) -> (11.0157, -99.2929)
  line L65 (11.0157, -99.2929) -> (-32.1178, -56.1594)
  line L66 (-32.1178, -56.1594) -> (6.8605, -17.1811)
  line L67 (6.8605, -17.1811) -> (-2.8334, -45.2225)
  line L68 (80.7737, -148.5837) -> (90.8281, -158.6381)
  line L69 (90.8281, -158.6381) -> (101.6485, -154.9105)
  line L70 (101.6485, -154.9105) -> (106.6034, -156.1112)
  line L71 (106.6034, -156.1112) -> (107.219, -156.2849)
  arc A16 (108.6531, -156.7089) -> (107.219, -156.2849) centre (83.2615, -239.9478) ccw
  line L72 (108.6531, -156.7089) -> (120.2894, -168.3453)
  line L73 (120.2894, -168.3453) -> (143.4763, -160.3296)
  line L74 (143.4763, -160.3296) -> (147.74, -161.7293)
  line L75 (147.74, -161.7293) -> (110.5961, -198.8732)
  line L76 (110.5961, -198.8732) -> (70.5402, -158.8173)
  line L77 (70.5402, -158.8173) -> (80.7737, -148.5837)
  line L78 (107.9565, -32.0507) -> (137.7824, -2.2247)
  line L79 (137.7824, -2.2247) -> (167.6083, -32.0507)
  line L80 (167.6083, -32.0507) -> (137.7824, -61.8766)
  line L81 (137.7824, -61.8766) -> (107.9565, -32.0507)
  line L82 (69.9473, 4.4661) -> (171.5721, -97.1586)
  line L83 (70.8941, 7.6696) -> (174.8254, -96.2616)
  line L84 (74.4297, 11.2052) -> (178.3609, -92.7261)
  point P0 (0, 0)
  point P1 (141.2327, -55.5979)
  point P2 (142.6469, -57.0121)
  point P3 (112.821, -27.1862)
  point P4 (114.2352, -28.6004)
  dimension "d179" = 5
  dimension "d202" = 3
  dimension "d210" = 16.7685
  dimension "d99" = 2
  dimension "d100" = 2
  dimension "d101" = 2
  dimension "d102" = 2
  dimension "d103" = 2
  dimension "d104" = 5
  constraints: 72 end point, 4 point on circle, 2 centre point, 1 parallel, 36 other
  measures "d99" distance between parallel lines of L34 L49
  measures "d100" distance between parallel lines of L19 L54
  measures "d101" distance between parallel lines of L43 L59
  measures "d102" distance between parallel lines of L24 L68
  measures "d103" distance between parallel lines of L13 L78
  measures "d104" distance between parallel lines of L83 L84
extrude "Extrusion23" add sketch "Sketch23" along normal blind 3 contours L12 L13 L84 L78 L79 L80 L15 | L49 L50 L51 L52 L53 | L54 L55 L56 L57 L58 | L59 A15 L60 L61 L62 L63 L64 L65 L66 L67 | L68 L69 L70 L71 A16 L72 L73 L74 L75 L76 L77
chamfer "Chamfer3" distance 3 angle 45 2 edges at (-141.9398, -56.305, -3) (-113.5281, -27.8933, -3)
sketch "Sketch24" plane through (-0.9798, 0.9798, -25.5) normal (0.7071068, 0.7071068, 0) x (-0.7071068, 0.7071068, 0)
  line L0 (37.1447, -109.0443) -> (-42.2248, 13.4196)
  line L1 (37.5643, -108.7723) -> (-41.8052, 13.6915)
  line L2 (-8.6834, 22.5) -> (-63.807, 22.5) projected
  line L3 (-28.486, 22.9196) -> (-42.4968, 13.8391)
  line L4 (-41.8052, 13.6915) -> (-39.0859, 9.4956)
  line L5 (-39.0859, 9.4956) -> (-25.4489, 18.3338)
  line L6 (-39.2335, 8.8041) -> (-42.2248, 13.4196)
  line L7 (-41.5333, 13.2719) -> (-27.9421, 22.0804)
  line L8 (-24.9051, 17.4947) -> (-39.3812, 8.1126)
  line L9 (-39.3812, 8.1126) -> (-42.6444, 13.1476)
  line L10 (-24.9051, 17.4947) -> (-25.4489, 18.3338)
  line L11 (-27.9421, 22.0804) -> (-28.486, 22.9196)
  line L12 (-39.0859, 9.4956) -> (-38.6663, 9.7676)
  line L13 (-39.3812, 8.1126) -> (-42.9163, 13.5672)
  line L14 (-42.9163, 13.5672) -> (-42.4968, 13.8391)
  line L15 (-39.0859, 9.4956) -> (-41.5333, 13.2719)
  line L16 (127.9704, 12.8461) -> (103.7728, -22.207)
  line L17 (127.9704, 12.8461) -> (127.9704, 39.3953)
  line L18 (127.9704, 12.8461) -> (127.9704, -5.4479)
  line L19 (124.4296, 8.6078) -> (127.2747, 12.7194)
  line L20 (127.9704, 12.8461) -> (124.8408, 8.3233)
  line L21 (127.2747, 12.7194) -> (126.8636, 13.0039)
  line L22 (110.8268, 17.4125) -> (124.5563, 7.9121)
  line L23 (124.7141, 9.019) -> (111.3958, 18.2349)
  line L24 (127.2747, 12.7194) -> (113.9116, 21.9663)
  line L25 (114.4806, 22.7887) -> (128.6661, 12.9727)
  line L26 (114.4806, 22.7887) -> (113.9116, 21.9663)
  line L27 (111.3958, 18.2349) -> (110.8268, 17.4125)
  line L28 (119.0075, -0.9854) -> (125.2519, 8.0388)
  line L29 (87.2319, 21.0024) -> (85.5512, 21.5755)
  line L30 (127.2747, 12.7194) -> (124.7141, 9.019)
  line L31 (124.9674, 7.6276) -> (124.5563, 7.9121)
  line L32 (114.4806, 22.7887) -> (127.7739, 28.2597)
  line L33 (124.9674, 7.6276) -> (132.7358, 18.854)
  line L34 (128.6661, 12.9727) -> (144.5653, 19.5162)
  line L35 (119.8383, 34.422) -> (126.3818, 18.5228) construction
  line L36 (128.6661, 12.9727) -> (118.6576, -1.491)
  line L37 (124.9674, 7.6276) -> (124.9473, -10.8779)
  point P0 (-1.3856, 25.5)
  point P1 (-28.2141, 22.5)
  point P2 (-29.1334, 22.5)
  point P3 (124.9486, 7.728)
  point P4 (124.1304, 8.5713)
  point P5 (124.7141, 9.019)
  point P6 (124.9674, 7.6276)
  point P7 (125.2519, 8.0388)
  dimension "d110" = 0.5
  dimension "d112" = 5
  dimension "d116" = 0.5
  dimension "d167" = 34.618
  dimension "d170" = 57.053
  dimension "d171" = 90
  dimension "d172" = 32.947
  dimension "d173" = 34.62
  constraints: 74 end point, 6 point on line, 5 perpendicular, 3 parallel, 2 vertical, 1 collinear, 6 other
  measures "d110" distance between parallel lines of L0 L1
  measures "d112" distance of L1.end L4.end
  measures "d116" distance of L4.end L12.end
  measures "d167" angle of L18 L16
  measures "d170" angle of L25 L32
  measures "d171" angle of L34 L35
  measures "d172" angle of L34 L33
  measures "d173" angle of L37 L36
ref_plane "Work Plane9" through (28.3887, -28.3887, -12.2281) normal (0.3845744, -0.3845744, 0.8391693) x (0.7071068, 0.7071068, 0)